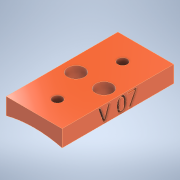
# Autodesk Inventor part: finderSupportPartV07
Saved by Autodesk Inventor 2021 (Build 250183000, 183)
## iProperties
Created: 2020-06-05
Part Number: finderSupportPartV07
Material: PC/ABS Plastic
Document SubType Name: Modeling
Designer: robst
Density: 0.357273 g/cm^3
Appearance: Smooth - Light Orange
Author: robst
Autodesk Inventor part; units mm, degrees
ref_plane "YZ Plane" through (0, 0, 0) normal (1, 0, 0) x (0, 1, 0)
ref_plane "XZ Plane" through (0, 0, 0) normal (0, 1, 0) x (-1, 0, 0)
ref_plane "XY Plane" through (0, 0, 0) normal (0, 0, 1) x (1, 0, 0)
sketch "Sketch1" plane through (0, 0, 0) normal (0, 0, 1) x (1, 0, 0)
  arc A0 (19.05, 73.7803) -> (-19.05, 73.7803) centre (0, 0) ccw
  line L0 (0, 85.2103) -> (19.05, 85.2103)
  line L1 (19.05, 85.2103) -> (19.05, 73.7803)
  line L2 (0, 76.2) -> (0, 85.2103) construction
  line L3 (0, 85.2103) -> (-19.05, 85.2103)
  line L4 (-19.05, 85.2103) -> (-19.05, 73.7803)
  dimension "d0" = 152.4
  dimension "d1" = 19.05
  dimension "d2" = 11.43
  constraints: 10 end point, 3 point on circle, 2 symmetric about line, 1 centre point, 1 coincident, 1 horizontal, 1 perpendicular, 1 vertical
  measures "d0" diameter of A0
  measures "d1" distance of L0.start L0.end
  measures "d2" distance of L0.end L1.end
extrude "Extrusion1" add sketch "Sketch1" along normal mid plane 76.2
sketch "Sketch23" plane through (-19.05, 85.2103, 38.1) normal (0, 1, 0) x (1, 0, 0)
  line L0 (38.1, 0) -> (0, 0) construction
  line L1 (19.05, 0) -> (19.05, 76.2) construction
  line L2 (0, 76.2) -> (38.1, 76.2) construction
  point P0 (19.05, 38.1)
  point P1 (19.05, 15.875)
  point P2 (19.05, 60.325)
  dimension "d183" = 15.875
  dimension "d184" = 15.875
  constraints: 2 end point, 2 midpoint, 2 point on line
  measures "d183" distance from line of L0 point (19.05, 15.875)
  measures "d184" distance from line of point (19.05, 60.325) L2
hole "Hole2" at (0, 85.2103, 22.225) at (0, 85.2103, -22.225) direction (0, -1, 0) diameter 5.1054 end through all counterbore diameter 6.5278 counterbore depth 7.874 clearance for "Hex Machine Screw" size "#10" standard "Ansi Unified Screw Threads"
sketch "Sketch24" plane through (-19.05, 85.2103, 38.1) normal (0, 1, 0) x (1, 0, 0)
  line L0 (0, 76.2) -> (0, 0) construction
  line L1 (0, 38.1) -> (38.1, 38.1) construction
  line L2 (38.1, 76.2) -> (38.1, 0) construction
  line L3 (38.1, 0) -> (0, 0) construction
  line L4 (19.05, 0) -> (19.05, 76.2) construction
  line L5 (0, 76.2) -> (38.1, 76.2) construction
  line L6 (28.575, 38.1) -> (28.575, 38.1) construction
  line L7 (34.29, 38.1) -> (34.29, 38.1)
  line L8 (22.86, 38.1) -> (22.86, 38.1)
  arc A0 (22.86, 38.1) -> (34.29, 38.1) centre (28.575, 38.1) ccw
  arc A1 (34.29, 38.1) -> (22.86, 38.1) centre (28.575, 38.1) ccw
  line L9 (9.525, 38.1) -> (9.525, 38.1) construction
  line L10 (15.24, 38.1) -> (15.24, 38.1)
  line L11 (3.81, 38.1) -> (3.81, 38.1)
  arc A2 (3.81, 38.1) -> (15.24, 38.1) centre (9.525, 38.1) ccw
  arc A3 (15.24, 38.1) -> (3.81, 38.1) centre (9.525, 38.1) ccw
  point P0 (19.05, 38.1)
  point P1 (28.575, 38.1)
  point P2 (9.525, 38.1)
  dimension "d192" = 9.525
  dimension "d194" = 9.525
  dimension "d195" = 19.05
  dimension "d199" = 11.43
  dimension "d200" = 11.43
  constraints: 20 end point, 8 point on circle, 8 tangent, 6 midpoint, 4 centre point, 3 parallel, 2 perpendicular, 2 point on line, 1 equal radius
  measures "d192" distance from line of point (28.575, 38.1) L4
  measures "d194" distance from line of point (9.525, 38.1) L4
  measures "d195" distance of point (28.575, 38.1) point (9.525, 38.1)
  measures "d200" distance between parallel lines of L11 L10
extrude "Extrusion8" cut sketch "Sketch24" against normal through all
sketch "Sketch25" plane through (19.05, 73.7803, 38.1) normal (1, 0, 0) x (0, 0, -1)
  line L0 (0, 11.43) -> (0, 0) construction
  line L1 (0, 5.715) -> (76.2, 5.715) construction
  line L2 (76.2, 11.43) -> (76.2, 0) construction
  line L3 (32.8705, 10.4775) -> (29.59, 0.9525)
  line L4 (29.59, 0.9525) -> (28.2238, 0.9525)
  line L5 (28.2238, 0.9525) -> (24.9433, 10.4775)
  line L6 (24.9433, 10.4775) -> (26.3018, 10.4775)
  line L7 (26.3018, 10.4775) -> (28.9416, 2.5657)
  line L8 (28.9416, 2.5657) -> (31.5815, 10.4775)
  line L9 (31.5815, 10.4775) -> (32.8705, 10.4775)
  spline S0 degree 2 poles (43.6382, 5.715) (43.6382, 3.1524) (42.1485, 0.7518) (40.597, 0.7518) knots 0 0 0 1 2 2 2
  spline S1 degree 2 poles (40.597, 0.7518) (39.0224, 0.7518) (37.5481, 3.1987) (37.5481, 5.7073) knots 0 0 0 1 2 2 2
  spline S2 degree 2 poles (37.5481, 5.7073) (37.5481, 8.2854) (39.0378, 10.6705) (40.597, 10.6705) knots 0 0 0 1 2 2 2
  spline S3 degree 2 poles (40.597, 10.6705) (42.1639, 10.6705) (43.6382, 8.2005) (43.6382, 5.715) knots 0 0 0 1 2 2 2
  spline S4 degree 2 poles (42.0019, 2.8127) (42.1871, 3.2836) (42.3415, 4.7347) (42.3415, 5.715) knots 0 0 0 1 2 2 2
  spline S5 degree 2 poles (42.3415, 5.715) (42.3415, 6.6953) (42.1871, 8.1387) (41.9941, 8.625) knots 0 0 0 1 2 2 2
  spline S6 degree 2 poles (41.9941, 8.625) (41.8012, 9.1113) (41.1296, 9.613) (40.597, 9.613) knots 0 0 0 1 2 2 2
  spline S7 degree 2 poles (40.597, 9.613) (40.0644, 9.613) (39.3775, 9.1113) (39.1768, 8.6096) knots 0 0 0 1 2 2 2
  spline S8 degree 2 poles (39.1768, 8.6096) (38.9838, 8.1233) (38.8449, 6.6413) (38.8449, 5.7073) knots 0 0 0 1 2 2 2
  spline S9 degree 2 poles (38.8449, 5.7073) (38.8449, 4.7038) (38.9684, 3.3608) (39.1691, 2.8359) knots 0 0 0 1 2 2 2
  spline S10 degree 2 poles (39.1691, 2.8359) (39.3543, 2.3419) (40.0413, 1.8093) (40.597, 1.8093) knots 0 0 0 1 2 2 2
  spline S11 degree 2 poles (40.597, 1.8093) (41.1219, 1.8093) (41.8089, 2.311) (42.0019, 2.8127) knots 0 0 0 1 2 2 2
  line L10 (50.8399, 9.0495) -> (46.718, 0.9525)
  line L11 (46.718, 0.9525) -> (45.3595, 0.9525)
  line L12 (45.3595, 0.9525) -> (49.7129, 9.3583)
  line L13 (49.7129, 9.3583) -> (44.7961, 9.3583)
  line L14 (44.7961, 9.3583) -> (44.7961, 10.4775)
  line L15 (44.7961, 10.4775) -> (50.8399, 10.4775)
  line L16 (50.8399, 10.4775) -> (50.8399, 9.0495)
  point P0 (38.1, -73.7803)
  constraints: 2 end point, 2 midpoint, 1 horizontal
extrude "Extrusion9" cut sketch "Sketch25" against normal blind 2.54
equation "\"d51\" = 0.125 * Sketch8_Pitch"
equation "\"Sketch8_Pitch\" = 0.79375"
equation "\"d53\" = 60deg"
equation "\"d72\" = 0.125 * Sketch10_Pitch"
equation "\"Sketch10_Pitch\" = 0.79375"
equation "\"d74\" = 60deg"
equation "\"d93\" = 0.125 * Sketch12_Pitch"
equation "\"Sketch12_Pitch\" = 0.79375"
equation "\"d95\" = 60deg"
equation "\"d114\" = 0.125 * Sketch14_Pitch"
equation "\"Sketch14_Pitch\" = 0.79375"
equation "\"d116\" = 60deg"
equation "\"d135\" = 0.125 * Sketch16_Pitch"
equation "\"Sketch16_Pitch\" = 0.79375"
equation "\"d137\" = 60deg"
equation "\"d156\" = 0.125 * Sketch18_Pitch"
equation "\"Sketch18_Pitch\" = 0.79375"
equation "\"d158\" = 60deg"
body "Solid1"
